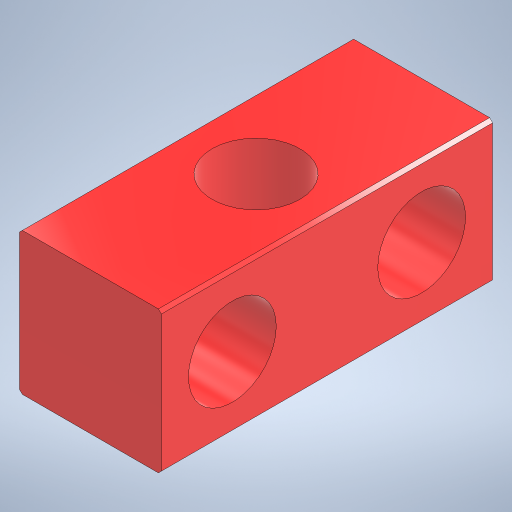
# Autodesk Inventor part: Nut Strip
Saved by Autodesk Inventor 2023.2 (Build 272271000, 271)
## iProperties
Created: 2024-01-21
Part Number: Nut Strip
Material: Aluminum 6061
Document SubType Name: Modeling
Designer: Nathan Cai
Density: 2.7 g/cm^3
Appearance: Light Red
Author: Nathan Cai
Autodesk Inventor part; units mm, degrees
ref_plane "YZ Plane" through (0, 0, 0) normal (1, 0, 0) x (0, 1, 0)
ref_plane "XZ Plane" through (0, 0, 0) normal (0, 1, 0) x (-1, 0, 0)
ref_plane "XY Plane" through (0, 0, 0) normal (0, 0, 1) x (1, 0, 0)
sketch "Sketch1" plane through (0, 0, 0) normal (0, 0, 1) x (1, 0, 0)
  line L0 (-2.3812, -2.3813) -> (2.3813, -2.3813)
  line L1 (2.3813, -2.3813) -> (2.3812, 2.3812)
  line L2 (2.3812, 2.3812) -> (-2.3813, 2.3812)
  line L3 (-2.3813, 2.3812) -> (-2.3812, -2.3813)
  line L4 (-2.3812, -2.3813) -> (2.3812, 2.3812) construction
  line L5 (2.3813, -2.3813) -> (-2.3813, 2.3812) construction
  point P0 (0, 0)
  dimension "d0" = 4.7625
  dimension "d1" = 4.7625
  constraints: 12 end point, 2 midpoint, 2 parallel, 1 horizontal, 1 perpendicular
  measures "d0" distance of L2.end L1.end
  measures "d1" distance of L1.end L0.end
extrude "Extrusion1" add sketch "Sketch1" along normal blind 11.1125
sketch "Sketch2" plane through (-2.3813, 2.3812, 0) normal (0, 1, 0) x (1, 0, 0)
  line L0 (2.3813, 0) -> (2.3813, -11.1125) construction
  line L1 (4.7625, -11.1125) -> (0, -11.1125) projected
  circle A0 centre (2.3813, -5.5563) radius 1.4732
  circle A1 centre (2.3813, -11.9062) radius 1.4732
  circle A2 centre (2.3813, -18.2563) radius 1.4732
  circle A3 centre (2.3813, -24.6063) radius 1.4732
  circle A4 centre (2.3813, -29.3688) radius 1.4493 construction
  line L2 (4.7625, 0) -> (0, 0) projected
  dimension "d4" = 2.9464
  dimension "d7" = 6.35
  dimension "d12" = 4.7625
  dimension "d13" = 5.5563
  constraints: 5 centre point, 2 end point, 2 midpoint, 1 point on line, 1 vertical, 6 other
  measures "d4" diameter of A0
  measures "d7" distance of A0.centre A1.centre
  measures "d12" distance of A3.centre A4.centre
  measures "d13" distance from line of L2 A0.centre
extrude "Extrusion2" cut sketch "Sketch2" against normal through all contours A0 | A2 | A3
sketch "Sketch3" plane through (2.3813, -2.3813, 0) normal (1, 0, 0) x (0, 0, -1)
  line L0 (0, 2.3813) -> (-11.1125, 2.3813) construction
  line L1 (-11.1125, 0) -> (-11.1125, 4.7625) projected
  circle A0 centre (-8.7312, 2.3813) radius 1.4732
  circle A1 centre (-2.3812, 2.3813) radius 1.4732
  circle A2 centre (3.9688, 2.3813) radius 1.4732
  circle A3 centre (10.3188, 2.3813) radius 1.4732
  dimension "d16" = 2.9464
  dimension "d17" = 2.3813
  dimension "d20" = 6.35
  constraints: 4 centre point, 2 end point, 1 horizontal, 1 midpoint, 1 point on line, 6 other
  measures "d16" diameter of A0
  measures "d17" distance from line of L1 A0.centre
  measures "d20" distance of A0.centre A1.centre
extrude "Extrusion3" cut sketch "Sketch3" against normal through all
chamfer "Chamfer1" distance 0.1 angle 45 4 edges at (-2.3813, 2.3812, 5.5563) (2.3812, 2.3812, 5.5563) (2.3813, -2.3813, 5.5563) (-2.3812, -2.3813, 5.5563)
equation "\"d1\" = d0"
body "Solid1"
